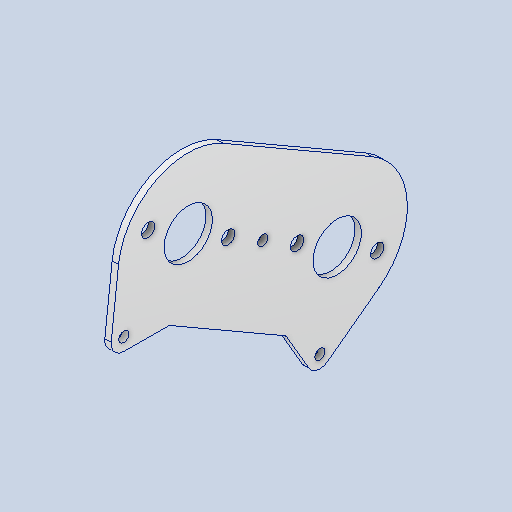
# Autodesk Inventor part: belt_liner_v5_Plate_15
Saved by Autodesk Inventor 2025.2 (Build 292293000, 293)
## iProperties
Created: 2025-03-06
Part Number: belt_liner_v5_Plate_15
Material: アルミニウム 6061
Document SubType Name: Modeling
Designer: haruy
Density: 2.7 g/cm^3
Appearance: アルミニウム - フラット
Author: haruy
Autodesk Inventor part; units mm, degrees
ref_plane "YZ Plane" through (0, 0, 0) normal (1, 0, 0) x (0, 1, 0)
ref_plane "XZ Plane" through (0, 0, 0) normal (0, 1, 0) x (-1, 0, 0)
ref_plane "XY Plane" through (0, 0, 0) normal (0, 0, 1) x (1, 0, 0)
derived "belt_liner_v5_Plate_14.ipt"
sketch "スケッチ1" plane through (300, 0, 0) normal (1, 0, 0) x (0, 1, 0)
  circle A0 centre (0, 0) radius 22.36 construction
  circle A1 centre (742.4003, -428.625) radius 23.875 construction
  line L0 (0, 0) -> (0, -985.832)
  line L1 (0, 0) -> (742.4003, -428.625) construction
  line L2 (-48.7433, -24.4258) -> (-56.2433, -37.4162)
  line L3 (-56.2433, -37.4162) -> (725.7777, -488.9162)
  line L4 (725.7777, -488.9162) -> (733.2777, -475.9258)
  line L5 (733.2777, -475.9258) -> (-48.7433, -24.4258) construction
  line L6 (-44.1225, 123.2584) -> (-44.1225, 123.2584)
  line L7 (0, -985.832) -> (0, 0)
  circle A2 centre (0, 0) radius 12.5
  circle A3 centre (0, 0) radius 15 construction
  line L8 (0, 0) -> (0, 0)
  circle A4 centre (0, 0) radius 24.06 construction
  line L9 (0, 0) -> (0, 0)
  line L10 (0, 0) -> (0, 0)
  line L11 (-48.7433, -24.4258) -> (-46.2433, -20.0957)
  circle A5 centre (742.4003, -428.625) radius 5 construction
  line L12 (733.2777, -475.9258) -> (707.2969, -460.9258)
  line L13 (707.2969, -460.9258) -> (709.7969, -456.5957)
  line L14 (709.7969, -456.5957) -> (735.7777, -471.5957)
  line L15 (735.7777, -471.5957) -> (733.2777, -475.9258)
  circle A6 centre (738.0702, -426.125) radius 5.1
  line L16 (742.4003, -428.625) -> (509.0943, -293.9257)
  circle A7 centre (759.7208, -438.625) radius 5.1
  line L17 (740.6202, -421.7083) -> (762.2708, -434.2083)
  line L18 (735.5202, -430.5417) -> (757.1708, -443.0417)
  circle A8 centre (742.4003, -428.625) radius 22.175 construction
  circle A9 centre (738.0702, -426.125) radius 10.1 construction
  circle A10 centre (759.7208, -438.625) radius 10.1 construction
  line L19 (743.1202, -417.3781) -> (764.7708, -429.8781) construction
  line L20 (733.0202, -434.8719) -> (754.6708, -447.3719) construction
  line L21 (743.1202, -417.3781) -> (730.6598, -410.1842) construction
  line L22 (729.3233, -421.075) -> (734.3733, -412.3281) construction
  line L23 (764.7708, -429.8781) -> (770.9335, -433.4362) construction
  line L24 (770.9335, -433.4362) -> (771.2695, -433.6302)
  line L25 (754.6708, -447.3719) -> (764.7708, -429.8781)
  line L26 (764.7708, -429.8781) -> (773.431, -434.8781)
  line L27 (773.431, -434.8781) -> (763.331, -452.3719)
  line L28 (763.331, -452.3719) -> (754.6708, -447.3719) construction
  circle A11 centre (725.8674, -468.7607) radius 1.5
  circle A12 centre (0, 0) radius 30 construction
  circle A13 centre (742.4003, -428.625) radius 6 construction
  circle A14 centre (0, 0) radius 24.06 construction
  circle A15 centre (0, 0) radius 24.06 construction
  circle A16 centre (742.4003, -428.625) radius 24.06
  line L29 (754.4303, -407.7884) -> (12.03, 20.8366) construction
  circle A17 centre (725.8592, -419.075) radius 4
  circle A18 centre (725.8592, -419.075) radius 1.5
  circle A19 centre (742.4003, -428.625) radius 18.525 construction
  circle A20 centre (748.9869, -417.4167) radius 4
  line L30 (737.4369, -437.4219) -> (742.4869, -428.675)
  circle A21 centre (748.9869, -417.4167) radius 1.5
  line L31 (734.3733, -412.3281) -> (737.8233, -406.3526) construction
  line L32 (737.8233, -406.3526) -> (776.881, -428.9026)
  line L33 (773.431, -434.8781) -> (776.881, -428.9026)
  line L34 (737.8233, -406.3526) -> (723.6503, -415.7402)
  circle A22 centre (735.9869, -439.9333) radius 4
  circle A23 centre (735.9869, -439.9333) radius 1.5
  line L35 (720.8233, -435.7974) -> (759.881, -458.3474)
  line L36 (763.331, -452.3719) -> (759.881, -458.3474)
  line L37 (720.8233, -435.7974) -> (721.8667, -418.8295)
  circle A24 centre (717.2072, -463.7607) radius 1.5
  circle A25 centre (742.4003, -428.625) radius 34.06
  circle A26 centre (742.4869, -428.675) radius 8.5
  line L38 (-57.9836, -13.421) -> (-72.9836, -13.421)
  line L39 (-72.9836, -13.421) -> (-72.9836, -278.421)
  line L40 (-72.9836, -278.421) -> (-57.9836, -278.421)
  line L41 (-57.9836, -278.421) -> (-57.9836, -13.421)
  line L42 (327.0164, -263.421) -> (-72.9836, -263.421)
  line L43 (-72.9836, -263.421) -> (-72.9836, -278.421)
  line L44 (-72.9836, -278.421) -> (327.0164, -278.421)
  line L45 (327.0164, -278.421) -> (327.0164, -263.421)
  line L46 (297.0164, -263.421) -> (297.0164, -278.421)
  line L47 (327.0164, -278.421) -> (361.1893, -278.421)
  line L48 (361.1893, -278.421) -> (368.6893, -265.4306)
  line L49 (-207.9836, 176.579) -> (-227.9836, 176.579)
  line L50 (-227.9836, 176.579) -> (-227.9836, -413.421)
  line L51 (-227.9836, -413.421) -> (-207.9836, -413.421)
  line L52 (-207.9836, -413.421) -> (-207.9836, 176.579)
  line L53 (-51.4069, -263.5692) -> (-53.919, -273.2486)
  line L54 (-53.919, -273.2486) -> (703.31, -469.7727)
  line L55 (703.31, -469.7727) -> (705.822, -460.0934)
  line L56 (705.822, -460.0934) -> (-51.4069, -263.5692)
  circle A27 centre (0, 0) radius 24.06 construction
  line L57 (1412.7204, 281.579) -> (-606.6364, 281.579)
  line L58 (1185.5776, -518.421) -> (-909.402, -518.421)
  line L59 (9.7721, 46.9258) -> (885.3238, -458.5742) construction
  line L60 (885.3238, -458.5742) -> (892.8238, -445.5838)
  line L61 (892.8238, -445.5838) -> (17.2721, 59.9162)
  line L62 (17.2721, 59.9162) -> (9.7721, 46.9258)
  line L63 (32.4276, 51.1662) -> (872.4722, -433.8338)
  line L64 (872.4722, -433.8338) -> (876.2222, -427.3386)
  line L65 (876.2222, -427.3386) -> (36.1776, 57.6614)
  line L66 (36.1776, 57.6614) -> (32.4276, 51.1662)
  line L67 (36.1776, 57.6614) -> (94.8941, 23.7614)
  line L68 (94.8941, 23.7614) -> (97.6441, 28.5245)
  line L69 (97.6441, 28.5245) -> (38.9276, 62.4245)
  line L70 (38.9276, 62.4245) -> (36.1776, 57.6614)
  circle A28 centre (218.0519, 108.5407) radius 120
  line L71 (77.0164, 123.579) -> (57.0164, 123.579)
  line L72 (57.0164, 123.579) -> (57.0164, 103.579)
  line L73 (57.0164, 103.579) -> (77.0164, 103.579)
  line L74 (77.0164, 103.579) -> (77.0164, 123.579)
  line L75 (218.0519, 108.5407) -> (186.9936, 224.4518)
  line L76 (218.0519, 108.5407) -> (102.1408, 77.4824)
  line L77 (218.0519, 108.5407) -> (158.0519, 4.6177)
  line L78 (189.9936, 229.648) -> (99.1408, 72.2863)
  line L79 (99.1408, 72.2863) -> (93.9447, 75.2863)
  line L80 (93.9447, 75.2863) -> (184.7975, 232.648)
  line L81 (184.7975, 232.648) -> (189.9936, 229.648)
  line L82 (184.7975, 232.648) -> (181.7975, 227.4518)
  line L83 (181.7975, 227.4518) -> (177.4674, 229.9518)
  line L84 (177.4674, 229.9518) -> (180.4674, 235.148)
  line L85 (180.4674, 235.148) -> (184.7975, 232.648)
  line L86 (93.9447, 75.2863) -> (96.9447, 80.4824)
  line L87 (96.9447, 80.4824) -> (92.6146, 82.9824)
  line L88 (92.6146, 82.9824) -> (89.6146, 77.7863)
  line L89 (89.6146, 77.7863) -> (93.9447, 75.2863)
  line L90 (77.0164, 123.579) -> (117.0164, 123.579)
  line L91 (117.0164, 123.579) -> (117.0164, 103.579)
  line L92 (117.0164, 103.579) -> (77.0164, 103.579)
  line L93 (77.0164, 103.579) -> (77.0164, 123.579)
  circle A29 centre (218.0519, 108.5407) radius 132.0681
  line L94 (103.6776, 174.5748) -> (38.9276, 62.4245)
  line L95 (32.4276, 51.1662) -> (11.6951, 15.2564) construction
  line L96 (11.6951, 15.2564) -> (20.3553, 10.2564) construction
  line L97 (20.3553, 10.2564) -> (41.0878, 46.1662) construction
  line L98 (41.0878, 46.1662) -> (32.4276, 51.1662)
  line L99 (152.0179, -5.8336) -> (158.0519, 4.6177)
  line L100 (152.0179, -5.8336) -> (20.3553, 10.2564) construction
  line L101 (74.8121, 3.6014) -> (78.3121, 9.6636)
  line L102 (78.3121, 9.6636) -> (92.5711, 1.4312)
  line L103 (181.7975, 227.4518) -> (154.2911, 210.1998)
  line L104 (96.9447, 80.4824) -> (98.1322, 112.9297)
  line L105 (99.1408, 72.2863) -> (116.3929, 44.7799)
  line L106 (-324.9836, 281.579) -> (-324.9836, -518.421)
  line L107 (1175.0164, 281.579) -> (1175.0164, -518.421)
  line L108 (17.2721, 59.9162) -> (9.7721, 46.9258)
  line L109 (9.7721, 46.9258) -> (-3.2183, 54.4258)
  line L110 (-3.2183, 54.4258) -> (4.2817, 67.4162)
  line L111 (4.2817, 67.4162) -> (17.2721, 59.9162)
  line L112 (-3.2183, 54.4258) -> (-5.7183, 50.0957)
  line L113 (-5.7183, 50.0957) -> (22.4276, 33.8457)
  line L114 (22.4276, 33.8457) -> (24.9276, 38.1758)
  line L115 (24.9276, 38.1758) -> (-3.2183, 54.4258)
  line L116 (-48.7433, -24.4258) -> (-46.2433, -20.0957)
  line L117 (-46.2433, -20.0957) -> (5.7183, -50.0957) construction
  line L118 (5.7183, -50.0957) -> (3.2183, -54.4258) construction
  line L119 (3.2183, -54.4258) -> (-48.7433, -24.4258) construction
  line L120 (789.6086, -403.313) -> (798.2689, -408.313)
  line L121 (798.2689, -408.313) -> (785.0364, -431.2324)
  line L122 (785.0364, -431.2324) -> (776.3761, -426.2324)
  line L123 (776.3761, -426.2324) -> (789.6086, -403.313)
  line L124 (885.3238, -458.5742) -> (882.8238, -462.9043)
  line L125 (882.8238, -462.9043) -> (856.843, -447.9043)
  line L126 (856.843, -447.9043) -> (859.343, -443.5742)
  line L127 (859.343, -443.5742) -> (885.3238, -458.5742)
  line L128 (7.6071, 48.1758) -> (11.9372, 45.6758)
  line L129 (11.9372, 45.6758) -> (19.4372, 58.6662)
  line L130 (19.4372, 58.6662) -> (15.1071, 61.1662)
  line L131 (15.1071, 61.1662) -> (7.6071, 48.1758)
  line L132 (19.4372, 58.6662) -> (14.4372, 50.0059)
  line L133 (14.4372, 50.0059) -> (24.8295, 44.0059)
  line L134 (24.8295, 44.0059) -> (29.8295, 52.6662)
  line L135 (29.8295, 52.6662) -> (19.4372, 58.6662)
  line L136 (931.2231, -485.0742) -> (935.5533, -487.5742)
  line L137 (935.5533, -487.5742) -> (951.5533, -459.8614)
  line L138 (951.5533, -459.8614) -> (947.2231, -457.3614)
  line L139 (947.2231, -457.3614) -> (931.2231, -485.0742)
  line L140 (944.4731, -462.1245) -> (934.9731, -478.579)
  line L141 (934.9731, -478.579) -> (919.3847, -469.579)
  line L142 (919.3847, -469.579) -> (928.8847, -453.1245)
  line L143 (928.8847, -453.1245) -> (944.4731, -462.1245)
  line L144 (924.1347, -461.3518) -> (939.7231, -470.3518)
  line L145 (926.6347, -457.0216) -> (921.6347, -465.6819)
  line L146 (921.6347, -465.6819) -> (882.6635, -443.1819)
  line L147 (882.6635, -443.1819) -> (887.6635, -434.5216)
  line L148 (887.6635, -434.5216) -> (926.6347, -457.0216)
  line L149 (888.9135, -432.3566) -> (881.4135, -445.347)
  line L150 (881.4135, -445.347) -> (874.4853, -441.347)
  line L151 (874.4853, -441.347) -> (881.9853, -428.3566)
  line L152 (881.9853, -428.3566) -> (888.9135, -432.3566)
  line L153 (31.0795, 54.8313) -> (23.5795, 41.8409)
  line L154 (23.5795, 41.8409) -> (30.5077, 37.8409)
  line L155 (30.5077, 37.8409) -> (38.0077, 50.8313)
  line L156 (38.0077, 50.8313) -> (31.0795, 54.8313)
  line L157 (16.9372, 54.3361) -> (27.3295, 48.3361)
  circle A30 centre (4.192, 47.2607) radius 1.25
  circle A31 centre (12.8522, 42.2607) radius 1.25
  line L158 (17.2721, 59.9162) -> (9.7721, 46.9258)
  line L159 (885.3238, -458.5742) -> (882.8238, -462.9043)
  line L160 (882.8238, -462.9043) -> (933.0533, -491.9043)
  line L161 (933.0533, -491.9043) -> (935.5533, -487.5742)
  line L162 (935.5533, -487.5742) -> (885.3238, -458.5742)
  line L163 (375.0164, 281.579) -> (375.0164, -518.421)
  line L164 (38.9276, 62.4245) -> (41.4276, 66.7546)
  line L165 (41.4276, 66.7546) -> (100.1441, 32.8546)
  line L166 (100.1441, 32.8546) -> (97.6441, 28.5245)
  line L167 (97.6441, 28.5245) -> (38.9276, 62.4245)
  line L168 (97.7242, 18.6633) -> (115.0447, 8.6633)
  line L169 (115.0447, 8.6633) -> (117.5447, 12.9934)
  line L170 (117.5447, 12.9934) -> (100.2242, 22.9934)
  line L171 (100.2242, 22.9934) -> (97.7242, 18.6633)
  line L172 (116.2947, 10.8284) -> (98.9742, 20.8284)
  line L173 (327.0164, -263.421) -> (335.2086, -263.421)
  line L174 (335.2086, -263.421) -> (342.7086, -250.4306)
  line L175 (-48.7433, -24.4258) -> (-56.2433, -37.4162)
  line L176 (-56.2433, -37.4162) -> (-77.8939, -24.9162)
  line L177 (-77.8939, -24.9162) -> (-70.3939, -11.9258)
  line L178 (-70.3939, -11.9258) -> (-48.7433, -24.4258)
  line L179 (-207.9836, -73.421) -> (-72.9836, -73.421) construction
  line L180 (-72.9836, -73.421) -> (-72.9836, -93.421)
  line L181 (-72.9836, -93.421) -> (-207.9836, -93.421) construction
  line L182 (-207.9836, -93.421) -> (-207.9836, -73.421)
  line L183 (-72.9836, -198.421) -> (-207.9836, -198.421) construction
  line L184 (-207.9836, -198.421) -> (-207.9836, -218.421)
  line L185 (-207.9836, -218.421) -> (-72.9836, -218.421) construction
  line L186 (-72.9836, -218.421) -> (-72.9836, -198.421)
  line L187 (-227.9836, -118.421) -> (-207.9836, -118.421)
  circle A32 centre (-30.1728, -32.2607) radius 1.25 construction
  circle A33 centre (-12.8522, -42.2607) radius 1.25 construction
  line L188 (-5.7183, 50.0957) -> (-46.2433, -20.0957)
  circle A34 centre (44.6769, 5.3827) radius 15 construction
  circle A35 centre (17.6769, -41.3827) radius 15 construction
  circle A36 centre (44.6769, 5.3827) radius 22
  circle A37 centre (17.6769, -41.3827) radius 22
  circle A38 centre (31.1769, -18) radius 3 construction
  line L189 (44.6769, 5.3827) -> (17.6769, -41.3827) construction
  circle A39 centre (26.7448, 25.5678) radius 3 construction
  circle A40 centre (-8.77, -35.9456) radius 3 construction
  circle A41 centre (866.7533, -450.7393) radius 1.25
  circle A42 centre (875.4135, -455.7393) radius 1.25
  circle A43 centre (994.8767, -339.9593) radius 120
  line L190 (278.0519, 212.4638) -> (1054.8767, -236.0362)
  line L191 (-207.9836, -118.421) -> (1175.0164, -118.421)
  line L192 (-227.9836, -283.421) -> (-207.9836, -283.421)
  line L193 (-72.9836, -68.421) -> (-92.9836, -68.421)
  line L194 (-92.9836, -68.421) -> (-92.9836, -88.421)
  line L195 (-92.9836, -88.421) -> (-72.9836, -88.421)
  line L196 (-72.9836, -88.421) -> (-72.9836, -68.421)
  line L197 (-72.9836, -218.421) -> (-92.9836, -218.421)
  line L198 (-92.9836, -218.421) -> (-92.9836, -238.421)
  line L199 (-92.9836, -238.421) -> (-72.9836, -238.421)
  line L200 (-72.9836, -238.421) -> (-72.9836, -218.421)
  circle A44 centre (-28.7272, -34.6374) radius 15
  circle A45 centre (26.7448, 25.5678) radius 1.6
  circle A46 centre (31.1769, -18) radius 1.6
  circle A47 centre (-8.77, -35.9456) radius 1.6
  circle A48 centre (44.6769, 5.3827) radius 7.6
  circle A49 centre (44.6769, 5.3827) radius 14.5
  circle A50 centre (37.4269, -7.1747) radius 2.1
  circle A51 centre (51.9269, 17.9401) radius 2.1
  circle A52 centre (17.6769, -41.3827) radius 7.6
  circle A53 centre (17.6769, -41.3827) radius 14.5
  circle A54 centre (24.9269, -28.8253) radius 2.1
  circle A55 centre (10.4269, -53.9401) radius 2.1
  circle A56 centre (-28.7272, -34.6374) radius 6.1
  circle A57 centre (-28.7272, -34.6374) radius 9
  circle A58 centre (-21.5807, -40.1081) radius 1.6
  circle A59 centre (-35.8736, -29.1667) radius 1.6
  circle A60 centre (26.7448, 25.5678) radius 4
  circle A61 centre (31.1769, -18) radius 4
  circle A62 centre (-8.77, -35.9456) radius 4
  line L201 (27.3403, 29.5233) -> (27.3403, 29.5233)
  line L202 (27.2027, 29.5415) -> (47.195, 27.2381)
  line L203 (63.7295, -5.6173) -> (36.7295, -52.3827)
  line L204 (22.7449, 25.5813) -> (22.677, 5.4568)
  line L205 (25.6244, 16.3827) -> (-1.3756, -30.3827)
  line L206 (17.5561, -19.383) -> (-28.8095, -19.6376) construction
  line L207 (-33.0766, -48.993) -> (11.2977, -62.4375) construction
  line L208 (-10.7816, -32.4883) -> (6.6128, -22.3673)
  line L209 (-11.9824, -38.329) -> (0.0086, -54.4911)
  line L210 (-92.9836, 143.579) -> (-112.9836, 143.579)
  line L211 (-112.9836, 143.579) -> (-112.9836, -340.421)
  line L212 (-112.9836, -340.421) -> (-92.9836, -340.421)
  line L213 (-92.9836, -340.421) -> (-92.9836, 143.579)
  line L214 (-98.6706, -321.2466) -> (-92.9836, -340.421)
  line L215 (-92.9836, -340.421) -> (762.3277, -86.7414)
  line L216 (762.3277, -86.7414) -> (756.6407, -67.567)
  line L217 (756.6407, -67.567) -> (-98.6706, -321.2466)
  line L218 (297.0164, -278.421) -> (282.0164, -278.421)
  line L219 (282.0164, -278.421) -> (282.0164, -293.421)
  line L220 (282.0164, -293.421) -> (297.0164, -293.421)
  line L221 (297.0164, -293.421) -> (297.0164, -278.421)
  line L222 (282.0164, -293.421) -> (267.0164, -293.421)
  line L223 (267.0164, -293.421) -> (267.0164, -210.9924)
  line L224 (267.0164, -210.9924) -> (282.0164, -210.9924)
  line L225 (282.0164, -210.9924) -> (282.0164, -293.421)
  line L226 (947.2231, -457.3614) -> (854.3308, -403.73)
  circle A63 centre (257.8891, 85.5407) radius 120
  point P0 (730.6598, -410.1842)
  point P1 (-65.4836, -23.421)
  point P2 (-65.4836, -270.921)
  point P3 (317.0164, -270.921)
  point P4 (307.0164, -270.921)
  point P5 (347.6105, -261.921)
  point P6 (356.2707, -266.921)
  point P7 (-42.9836, -270.921)
  point P8 (694.8867, -462.421)
  point P9 (57.0164, 113.579)
  point P10 (782.9924, -414.7727)
  point P11 (931.9289, -465.8518)
  point P12 (22.6968, 11.312)
  point P13 (1.5519, -25.312)
  point P14 (0, -54.4795)
  point P15 (274.5164, -220.9924)
extrude "押し出し1" add sketch "スケッチ1" against normal blind 2 contours L208 L205 L0 | L0 L205 A37 L209 A62 L208 | L205 L208 A37 L0 | L0 A37 L205 | A62 | L205 L204 A36 L203 A37 L208 | A37 L0 | L0 A37 | L205 A36 L204 | L204 A60 L202 A36 L205 | A60 | A36 | A49 A50 A51 | A53 A55 A54 | A61
fillet "フィレット1" radius 2 2 edges at (299, 22.6968, 11.312) (299, 1.5519, -25.312)
